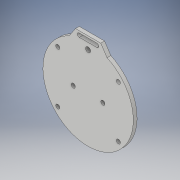
# Autodesk Inventor part: Back Plate
Saved by Autodesk Inventor 2018 (Build 220112000, 112)
## iProperties
Company: UNH Makerspace
Created: 2019-07-21
Part Number: Back Plate
Material: Generic
Document SubType Name: Modeling
Designer: Electro707
Density: 1 g/cm^3
Appearance: Default
Mass: 12.1057 g
Surface Area: 90.9921 cm^2
Volume: 12.1057 cm^3
Description: Back-plate for PCB
Engineer: Jamal Bouajjaj
Author: Electro707
Title: Tree Ornament - Back Plate
Revision Number: N/A
Autodesk Inventor part; units mm, degrees
ref_plane "YZ Plane" through (0, 0, 0) normal (1, 0, 0) x (0, 1, 0)
ref_plane "XZ Plane" through (0, 0, 0) normal (0, 1, 0) x (-1, 0, 0)
ref_plane "XY Plane" through (0, 0, 0) normal (0, 0, 1) x (1, 0, 0)
sketch "Sketch1" plane through (48, 0, 0) normal (0, 0, -1) x (-1, 0, 0)
  arc A0 (-15, 28.6843) -> (15, 28.6843) centre (0, -3.8157) ccw projected
  line L0 (-15, 28.6843) -> (-10, 36.1843) projected
  line L1 (0, 31.6843) -> (-7, 31.6843) projected
  arc A1 (-7, 34.6843) -> (-7, 31.6843) centre (-7, 33.1843) ccw projected
  line L2 (-10, 36.1843) -> (10, 36.1843) projected
  line L3 (10, 36.1843) -> (15, 28.6843) projected
  line L4 (0, 34.6843) -> (7, 34.6843) projected
  arc A2 (7, 31.6843) -> (7, 34.6843) centre (7, 33.1843) ccw projected
  line L5 (7, 31.6843) -> (0, 31.6843) projected
  circle A3 centre (24, 16.6843) radius 1.6 projected
  circle A4 centre (-24, 16.6843) radius 1.6 projected
  line L6 (-7, 34.6843) -> (0, 34.6843) projected
  circle A5 centre (24, -24.3157) radius 1.6 projected
  circle A6 centre (-24, -24.3157) radius 1.6 projected
  point P0 (48, 0)
extrude "Extrusion1" add sketch "Sketch1" along normal blind 3
sketch "Sketch2" plane through (48, 0, -3) normal (0, 0, -1) x (-1, 0, 0)
  line L0 (-20, 23.6843) -> (20, 23.6843) construction
  line L1 (20, 23.6843) -> (20, -31.3157) construction
  line L2 (20, -31.3157) -> (-20, -31.3157) construction
  line L3 (-20, -31.3157) -> (-20, 23.6843) construction
  circle A0 centre (11.7475, -3.8157) radius 1.65
  circle A1 centre (-11.7475, -3.8157) radius 1.65
  line L4 (0, -3.8157) -> (-11.7475, -3.8157) construction
  line L5 (0, -3.8157) -> (11.7475, -3.8157) construction
  circle A2 centre (24, 16.6843) radius 1.6 construction
  circle A3 centre (-24, 16.6843) radius 1.6 construction
  circle A4 centre (-24, -24.3157) radius 1.6 construction
  circle A5 centre (24, -24.3157) radius 1.6 construction
  line L6 (20, 23.6843) -> (24, 16.6843) construction
  line L7 (20, -31.3157) -> (24, -24.3157) construction
  line L8 (-20, 23.6843) -> (-24, 16.6843) construction
  line L9 (-20, -31.3157) -> (-24, -24.3157) construction
  circle A6 centre (0, 26.6843) radius 2
  line L10 (-20, 23.6843) -> (0, 26.6843) construction
  line L11 (0, 26.6843) -> (20, 23.6843) construction
  arc A7 (-15, 28.6843) -> (15, 28.6843) centre (0, -3.8157) ccw construction
  dimension "d2" = 55
  dimension "d3" = 40
  dimension "d4" = 3.3
  dimension "d5" = 23.495
  dimension "d8" = 4
  dimension "d9" = 3
  constraints: 24 end point, 5 equal length, 3 centre point, 3 horizontal, 2 parallel, 1 coincident, 1 equal radius, 1 perpendicular
  measures "d2" distance of L2.end L0.start
  measures "d3" distance of L0.start L0.end
  measures "d4" diameter of A1
  measures "d5" distance of L5.end L4.end
  measures "d8" diameter of A6
  measures "d9" vertical distance of L0.start L10.end
extrude "Extrusion2" cut sketch "Sketch2" against normal through all
body "Solid1"
